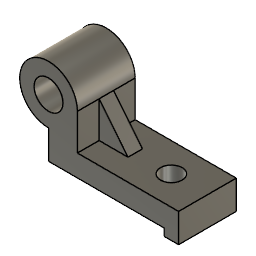
ISO 1 (Autodesk Fusion 360 design; units mm, degrees)
part number: 2025-12-08-12-07-30-035
Autodesk Fusion 360 part; units mm, degrees
sketch "Sketch1" plane through (0, 0, 0) normal (0, 1, 0) x (1, 0, 0)
  circle A0 centre (0, 0) radius 10
  line L0 (0, 40) -> (80, 40)
  line L1 (20, 0) -> (20, 25)
  line L2 (20, 25) -> (80, 25)
  arc A1 (0, 20) -> (20, 0) centre (0, 0) ccw
  line L3 (80, 25) -> (90, 25)
  line L4 (90, 25) -> (90, 45)
  line L5 (90, 45) -> (80, 45)
  line L6 (80, 45) -> (80, 40)
  line L7 (0, 20) -> (0, 40)
  dimension "d1" = 20
  dimension "d2" = 40
  dimension "d3" = 40
  dimension "d4" = 80
  dimension "d5" = 15
  dimension "d6" = 5
  dimension "d7" = 10
  constraint coincident A0.centre A1.centre
  constraint tangent L1 A1
  constraint vertical L1
  constraint horizontal L3
  constraint vertical L4
  constraint horizontal L5
  constraint vertical L6
  measures "d1" diameter of A0
  measures "d2" diameter of A1
  measures "d3" distance of A0.centre L0.start
  measures "d4" distance of L0.start L0.end
  measures "d5" distance of L0.end L2.end
  measures "d6" distance of L0.end L5.end
  measures "d7" distance of L4.end L5.end
extrude "Extrude1" add sketch "Sketch1" along normal mid plane 40
sketch "Sketch2" plane through (0, 0, 0) normal (0, 1, 0) x (1, 0, 0)
sketch "Sketch3" plane through (0, 0, -25) normal (0, 0, 1) x (-1, 0, 0)
  line L0 (-90, 20) -> (-90, -20)
  line L1 (-90, -20) -> (-20, -20)
  line L2 (-20, -20) -> (-20, 20)
  line L3 (-20, 20) -> (-90, 20)
  circle A0 centre (-65, 0) radius 7.5
  dimension "d10" = 15
  dimension "d11" = 25
  dimension "d12" = 20
  measures "d10" diameter of A0
  measures "d11" distance of L0 A0.centre
  measures "d12" distance of L1 A0.centre
extrude "Extrude2" cut sketch "Sketch3" against normal blind 40 contours A0
ref_plane "WorkPlane1" through (35, 0, -12.5) normal (0, -1, 0) x (-1, 0, 0)
sketch "Sketch4" plane through (0, 0, 0) normal (0, -1, 0) x (-1, 0, 0)
  line L0 (-20, 0) -> (-40, 25)
  line L1 (-20, 0) -> (-20, 25)
  line L2 (-20, 25) -> (-40, 25)
  constraint vertical L1
  constraint perpendicular L1 L2
extrude "Extrude3" add sketch "Sketch4" along normal mid plane 10
